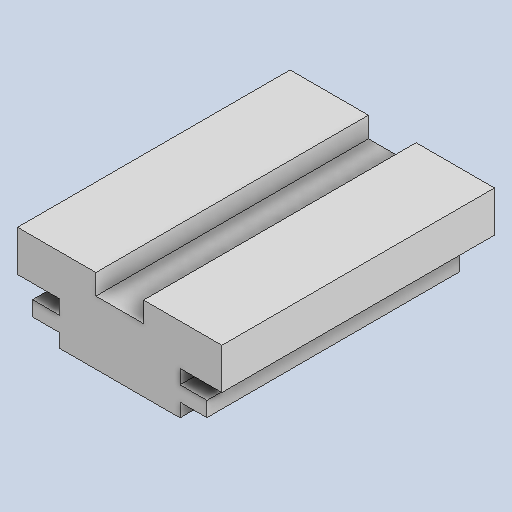
# Autodesk Inventor part: horok
Saved by Autodesk Inventor 2025 (Build 290162000, 162)
## iProperties
Created: 2025-09-19
Part Number: horok
Material: Generic
Document SubType Name: Modeling
Designer: Pravoslav
Density: 1 g/cm^3
Appearance: Default
Author: Pravoslav
Autodesk Inventor part; units mm, degrees
ref_plane "YZ Plane" through (0, 0, 0) normal (1, 0, 0) x (0, 1, 0)
ref_plane "XZ Plane" through (0, 0, 0) normal (0, 1, 0) x (-1, 0, 0)
ref_plane "XY Plane" through (0, 0, 0) normal (0, 0, 1) x (1, 0, 0)
sketch "Sketch1" plane through (0, 0, 0) normal (0, 1, 0) x (-1, 0, 0)
  line L0 (15, 20) -> (-15, 20)
  line L1 (-15, 20) -> (-15, -20)
  line L2 (-15, -20) -> (15, -20)
  line L3 (15, -20) -> (15, 20)
  line L4 (15, 20) -> (-15, -20) construction
  line L5 (-15, 20) -> (15, -20) construction
  point P0 (0, 0)
  dimension "d0" = 30
  dimension "d1" = 40
  constraints: 12 end point, 2 midpoint, 2 parallel, 1 horizontal, 1 perpendicular
  measures "d0" distance of L2.end L1.end
  measures "d1" distance of L1.end L0.end
extrude "Extrusion1" add sketch "Sketch1" along normal blind 3
sketch "Sketch2" plane through (0, 3, 0) normal (0, 1, 0) x (1, 0, 0)
  line L0 (-15, 20) -> (-15, -20) projected
  line L1 (15, 20) -> (-15, 20) projected
  line L2 (-15, -20) -> (-3.5, -20)
  line L3 (-3.5, -20) -> (-3.5, 20)
  line L4 (-3.5, 20) -> (-15, 20)
  line L5 (-15, 20) -> (-15, -20)
  line L6 (15, -20) -> (3.5, -20)
  line L7 (3.5, -20) -> (3.5, 20)
  line L8 (3.5, 20) -> (15, 20)
  line L9 (15, 20) -> (15, -20)
  point P0 (0, 0)
  dimension "d4" = 7
  dimension "d5" = 3.5
  dimension "d6" = 15
  constraints: 16 end point, 4 parallel, 3 point on line, 2 horizontal, 2 perpendicular
  measures "d4" distance between parallel lines of L7 L3
  measures "d5" distance from line of point (0, 0) L3
  measures "d6" distance from line of L9 point (0, 0)
extrude "Extrusion2" add sketch "Sketch2" along normal blind 3
sketch "Sketch3" plane through (0, 0, 0) normal (0, -1, 0) x (1, 0, 0)
  line L0 (15, -20) -> (-15, -20) projected
  line L1 (8.85, 20) -> (-8.85, 20)
  line L2 (-8.85, 20) -> (-8.85, -20)
  line L3 (-8.85, -20) -> (8.85, -20)
  line L4 (8.85, -20) -> (8.85, 20)
  line L5 (8.85, 20) -> (-8.85, -20) construction
  line L6 (-8.85, 20) -> (8.85, -20) construction
  point P0 (0, 0)
  dimension "d9" = 17.7
  constraints: 12 end point, 2 midpoint, 2 parallel, 1 horizontal, 1 perpendicular, 1 point on line
  measures "d9" distance between parallel lines of L2 L4
extrude "Extrusion3" add sketch "Sketch3" along normal blind 2.1
sketch "Sketch4" plane through (0, -2.1, 0) normal (0, -1, 0) x (1, 0, 0)
  line L0 (-8.85, -20) -> (-15, -20) projected
  line L1 (12.8, 20) -> (-12.8, 20)
  line L2 (-12.8, 20) -> (-12.8, -20)
  line L3 (-12.8, -20) -> (12.8, -20)
  line L4 (12.8, -20) -> (12.8, 20)
  line L5 (12.8, 20) -> (-12.8, -20) construction
  line L6 (-12.8, 20) -> (12.8, -20) construction
  line L7 (15, 20) -> (15, -20) projected
  line L8 (-12.8, -17) -> (12.8, -17)
  line L9 (8.85, -20) -> (8.85, 20) projected
  line L10 (8.85, -20) -> (8.85, -17)
  line L11 (-8.85, -20) -> (-8.85, -17)
  point P0 (0, 0)
  dimension "d12" = 2.2
  dimension "d15" = 3
  constraints: 18 end point, 6 point on line, 3 perpendicular, 2 midpoint, 2 parallel, 1 horizontal
  measures "d12" distance between parallel lines of L7 L4
  measures "d15" distance between parallel lines of L3 L8
extrude "Extrusion4" add sketch "Sketch4" along normal blind 2.2 contours L11 L8 L9 L3 | L8 L2 L1 L9 | L9 L1 L4 L8
sketch "Sketch5" plane through (0, -4.3, 0) normal (0, -1, 0) x (1, 0, 0)
  line L0 (-3.5, -20) -> (-15, -20) projected
  line L1 (8.85, 20) -> (-8.85, 20)
  line L2 (-8.85, 20) -> (-8.85, -20)
  line L3 (-8.85, -20) -> (8.85, -20)
  line L4 (8.85, -20) -> (8.85, 20)
  line L5 (8.85, 20) -> (-8.85, -20) construction
  line L6 (-8.85, 20) -> (8.85, -20) construction
  point P0 (0, 0)
  dimension "d16" = 17.7
  constraints: 12 end point, 2 midpoint, 2 parallel, 1 horizontal, 1 perpendicular, 1 point on line
  measures "d16" distance of L3.end L2.end
extrude "Extrusion5" add sketch "Sketch5" along normal blind 2
body "Solid1"
